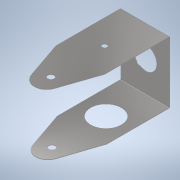
# Autodesk Inventor part: Frame
Saved by Autodesk Inventor 2020.3 (Build 243373000, 373)
## iProperties
Created: 2022-06-23
Part Number: Frame
Material: Steel, Alloy
Document SubType Name: Sheet Metal
Designer: karimi2
Density: 7.73 g/cm^3
Sheet Metal Rule: Default_mm
Appearance: Semi-Polished
Author: karimi2
Autodesk Inventor part; units mm, degrees
ref_plane "YZ Plane" through (0, 0, 0) normal (1, 0, 0) x (0, 1, 0)
ref_plane "XZ Plane" through (0, 0, 0) normal (0, 1, 0) x (-1, 0, 0)
ref_plane "XY Plane" through (0, 0, 0) normal (0, 0, 1) x (1, 0, 0)
sketch "Sketch1" plane through (0, 0, 0) normal (0, 0, 1) x (1, 0, 0)
  line L0 (-20, 90) -> (-20, 37.5)
  circle A0 centre (0, 13.2368) radius 2.6
  circle A1 centre (0, 57.5) radius 12.5
  line L1 (20, 90) -> (20, 38.2368)
  line L2 (-20, 90) -> (20, 90) construction
  line L3 (20, 90) -> (20, 140)
  line L4 (20, 140) -> (-20, 140) construction
  line L5 (-20, 140) -> (-20, 90)
  line L6 (20, 140) -> (20, 192.5)
  line L7 (-20, 140) -> (-20, 192.5)
  circle A2 centre (0, 172.5) radius 2
  circle A3 centre (0, 216.5) radius 2.6
  arc A4 (9.4595, 223.2432) -> (-9.4595, 223.2432) centre (0, 220) ccw
  line L8 (20, 192.5) -> (9.4595, 223.2432)
  line L9 (-20, 192.5) -> (-9.4595, 223.2432)
  circle A5 centre (0, 115) radius 9.5
  arc A6 (-9.4595, 6.7568) -> (9.4826, 6.825) centre (0, 10) ccw
  line L10 (-28, 0) -> (28, 0)
  line L11 (20, 38.2368) -> (9.4826, 6.825)
  line L12 (-20, 37.5) -> (-9.4595, 6.7568)
  line L13 (0, -46.3158) -> (0, 276.0526)
  point P0 (0, 0)
  point P1 (0, -0.2632)
  point P2 (0, 90)
  dimension "d0" = 52.5
  dimension "d1" = 13.5
  dimension "d2" = 5.2
  dimension "d5" = 25
  dimension "d7" = 50
  dimension "d8" = 40
  dimension "d10" = 52.5
  dimension "d11" = 32.5
  dimension "d12" = 4
  dimension "d13" = 24
  dimension "d14" = 5.2
  dimension "d15" = 20
  dimension "d41" = 19
  dimension "d42" = 25
  dimension "d47" = 20
  dimension "d48" = 25
  measures "d0" distance of L5.end L0.end
  measures "d1" distance of point (0, -0.263) A0.centre
  measures "d2" diameter of A0
  measures "d5" diameter of A1
  measures "d7" distance of L3.start L6.start
  measures "d8" distance of L6.start L7.start
  measures "d10" distance of L7.start L9.start
  measures "d11" distance from line of L4 A2.centre
  measures "d12" diameter of A2
  measures "d13" vertical distance of L8.start A3.centre
  measures "d14" diameter of A3
  measures "d15" diameter of A4
  measures "d41" diameter of A5
  measures "d42" distance of point (0, 90) A5.centre
  measures "d47" diameter of A6
  measures "d48" vertical distance of L1.end A0.centre
extrude "Plate1" add sketch "Sketch1" along normal mid plane 0.5 contours L5 L7 L9 A4 L13 A3 A2 A5 A1 A0 A6 L12 L0 | L13 A0 A1 A5 A2 A3 A4 L8 L6 L3 L1 L11 A6 | L13 A5 | A5 L13
sketch "Sketch4" plane through (0, 0, 0.25) normal (0, 0, 1) x (1, 0, 0)
  line L0 (-20, 90) -> (20, 90)
  line L1 (20, 192.5) -> (20, 38.2368) projected
  line L2 (-20, 140) -> (20, 140)
  point P0 (0, 0)
  dimension "d24" = 40
  dimension "d25" = 90
  dimension "d26" = 140
  constraints: 4 end point, 2 horizontal, 2 point on line
  measures "d24" distance of L0.start L0.end
  measures "d25" vertical distance of point (0, 0) L0.end
  measures "d26" vertical distance of point (0, 0) L2.end
fold "Fold1" angle 90 bend radius 0.5 thickness 0.5 k factor 0.44 line from (-20, 140, 0.25) to (20, 140, 0.25) line at bend end moving side (0, 1, 0) folds toward (0, 0, 1)
sketch "Sketch5" plane through (0, 0, 0.25) normal (0, 0, 1) x (1, 0, 0)
  line L0 (-20, 37.5) -> (-20, 138.869) projected
  line L1 (-20, 90) -> (20, 90)
  point P0 (0, 0)
  dimension "d33" = 40
  dimension "d34" = 90
  constraints: 2 end point, 1 horizontal, 1 point on line
  measures "d33" distance of L1.start L1.end
  measures "d34" vertical distance of point (0, 0) L1.end
fold "Fold2" angle 90 bend radius 0.5 thickness 0.5 k factor 0.44 line from (-20, 90, 0.25) to (20, 90, 0.25) line at bend start moving side (0, -1, 0) folds toward (0, 0, 1)
sketch "Sketch6" plane through (0, 0, -0.25) normal (0, 0, -1) x (-1, 0, 0)
  circle A0 centre (0, 115) radius 9.5
  line L0 (-20, 90) -> (20, 90) projected
  point P0 (0, 0)
  dimension "d43" = 25
  dimension "d44" = 19
  constraints: 1 centre point
  measures "d43" distance from line of L0 A0.centre
  measures "d44" diameter of A0
extrude "Extrusion2" cut sketch "Sketch6" against normal through all
equation "\"d23\" = Thickness"
equation "\"d27\" = BendReliefWidth"
equation "\"d28\" = BendReliefDepth"
equation "\"d29\" = MinimumRemnant"
equation "\"d30\" = TransitionRadius"
equation "\"d32\" = BendRadius"
equation "\"d35\" = BendReliefWidth"
equation "\"d36\" = BendReliefDepth"
equation "\"d37\" = MinimumRemnant"
equation "\"d38\" = TransitionRadius"
equation "\"d40\" = BendRadius"
equation "\"BendRadius\" = Thickness"
equation "\"BendReliefWidth\" = Thickness"
equation "\"BendReliefDepth\" = 0.5 * Thickness"
equation "\"CornerReliefSize\" = 4 * Thickness"
equation "\"MinimumRemnant\" = 2 * Thickness"
equation "\"TransitionRadius\" = BendRadius"
equation "\"JacobiRadiusSize\" = BendRadius"
equation "\"GapSize\" = Thickness"
equation "\"Thickness\" = 0.5"
body "Solid2"
